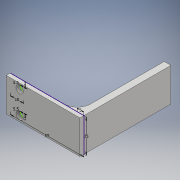
# Autodesk Inventor part: Camera_Wiper
Saved by Autodesk Inventor 2017 (Build 210142000, 142)
## iProperties
Created: 2017-01-15
Part Number: Camera_Wiper
Material: Generic
Document SubType Name: Modeling
Designer: willt
Density: 1 g/cm^3
Appearance: Default
Author: willt
Autodesk Inventor part; units mm, degrees
ref_plane "YZ Plane" through (0, 0, 0) normal (1, 0, 0) x (0, 1, 0)
ref_plane "XZ Plane" through (0, 0, 0) normal (0, 1, 0) x (-1, 0, 0)
ref_plane "XY Plane" through (0, 0, 0) normal (0, 0, 1) x (1, 0, 0)
sketch "Sketch1" plane through (0, 0, 0) normal (0, 1, 0) x (-1, 0, 0)
  line L0 (27.5, 12.5) -> (-27.5, 12.5)
  line L1 (-27.5, 12.5) -> (-27.5, -12.5)
  line L2 (-27.5, -12.5) -> (27.5, -12.5)
  line L3 (27.5, -12.5) -> (27.5, 12.5)
  line L4 (27.5, 12.5) -> (-27.5, -12.5) construction
  line L5 (-27.5, 12.5) -> (27.5, -12.5) construction
  line L6 (27.5, 0) -> (17.5, 0) construction
  line L7 (17.5, 12.5) -> (17.5, 8.5) construction
  line L8 (17.5, -12.5) -> (17.5, -8.5) construction
  circle A0 centre (17.5, 8.5) radius 2.75
  circle A1 centre (17.5, -8.5) radius 2.75
  line L9 (-27.5, 12.5) -> (-22.5, 12.5) construction
  line L10 (-22.5, 12.5) -> (-22.5, -12.5)
  point P0 (0, 0)
  dimension "d0" = 55
  dimension "d1" = 25
  dimension "d2" = 10
  dimension "d3" = 4
  dimension "d4" = 4
  dimension "d5" = 5.5
  dimension "d6" = 5.5
  dimension "d7" = 5
  constraints: 22 end point, 4 point on line, 3 midpoint, 3 perpendicular, 2 centre point, 2 coincident, 2 horizontal, 2 parallel, 1 vertical
  measures "d0" distance of L2.end L1.end
  measures "d1" distance of L1.end L0.end
  measures "d2" distance of L6.start L6.end
  measures "d3" distance of L7.start L7.end
  measures "d4" distance of L8.start L8.end
  measures "d5" diameter of A0
  measures "d6" diameter of A1
  measures "d7" distance of L0.end L9.end
extrude "Extrusion1" add sketch "Sketch1" against normal blind 3 contours L3 L2 L10 L0
extrude "Extrusion2" add sketch "Sketch1" against normal blind 3 contours L10 L2 L1 L0
extrude "Extrusion3" add sketch "Sketch1" along normal blind 65 contours L10 L2 L1 L0
sketch "Sketch2" plane through (0, 65, 0) normal (0, 1, 0) x (1, 0, 0)
  line L0 (27.5, -12.5) -> (-27.5, -12.5) construction
  line L1 (27.5, -12.5) -> (25, -12.5) construction
  line L2 (25, -12.5) -> (25, -10) construction
  line L3 (27.5, 12.5) -> (22.5, 12.5) construction
  line L4 (25, 12.5) -> (25, 10) construction
  circle A0 centre (25, -10) radius 0.75
  circle A1 centre (25, 10) radius 0.75
  point P0 (0, 0)
  dimension "d14" = 2.5
  dimension "d15" = 2.5
  dimension "d16" = 2.5
  dimension "d17" = 1.5
  dimension "d18" = 1.5
  constraints: 6 end point, 2 centre point, 2 coincident, 1 midpoint, 1 perpendicular, 1 point on line, 1 vertical
  measures "d14" distance of L0.start L1.end
  measures "d15" distance of L1.end L2.end
  measures "d16" distance of L4.start L4.end
  measures "d17" diameter of A0
  measures "d18" diameter of A1
extrude "Extrusion4" cut sketch "Sketch2" against normal blind 20
fillet "Fillet1" radius 10 1 edges at (22.5, 0, 0)
body "Solid1"
